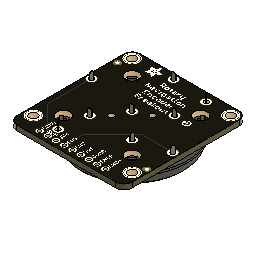
5221 ANO Rotary Encoder (Autodesk Fusion 360 design; units mm, degrees)
part number: MOUNTINGHOLE2.5
part number: FIDUCIAL_1MM
part number: ENCODER_ANO
Autodesk Fusion 360 part; units mm, degrees
sketch "sketch 280" plane through (0, 0, 0) normal (0, 0, 1) x (1, 0, 0)
  line L0 (17.78, -17.78) -> (17.78, 15.24)
  arc A0 (17.78, 15.24) -> (15.24, 17.78) centre (15.24, 15.24) ccw
  line L1 (15.24, 17.78) -> (-15.24, 17.78)
  arc A1 (-15.24, 17.78) -> (-17.78, 15.24) centre (-15.24, 15.24) ccw
  line L2 (-17.78, 15.24) -> (-17.78, -17.78)
  arc A2 (-17.78, -17.78) -> (-15.24, -20.32) centre (-15.24, -17.78) ccw
  line L3 (-15.24, -20.32) -> (15.24, -20.32)
  arc A3 (15.24, -20.32) -> (17.78, -17.78) centre (15.24, -17.78) ccw
extrude "Board" add sketch "sketch 280" along normal blind 1.57 makes body 1 in component "Board"
sketch "sketch 711" plane through (0, 0, 0) normal (0, 0, 1) x (1, 0, 0)
  line L0 (-2, -2) -> (2, -2)
  line L1 (2, -2) -> (2, 2)
  line L2 (2, 2) -> (-2, 2)
  line L3 (-2, 2) -> (-2, -2)
extrude "MOUNTINGHOLE_2.5_PLATED" add sketch "sketch 711" along normal blind 0.1 separate body makes body 2 in component "MOUNTINGHOLE_2.5_PLATED"
sketch "sketch 850" plane through (0, 0, 0) normal (0, 0, 1) x (1, 0, 0)
  line L0 (-0.75, -0.75) -> (0.75, -0.75)
  line L1 (0.75, -0.75) -> (0.75, 0.75)
  line L2 (0.75, 0.75) -> (-0.75, 0.75)
  line L3 (-0.75, 0.75) -> (-0.75, -0.75)
extrude "FIDUCIAL_1MM" add sketch "sketch 850" along normal blind 0.1 separate body makes body 3 in component "FIDUCIAL_1MM"
sketch "sketch 981" plane through (0, 0, 0) normal (0, 0, 1) x (1, 0, 0)
  line L0 (0.016, 0.016) -> (3.794, 0.016)
  line L1 (3.794, 0.016) -> (3.794, 3.794)
  line L2 (3.794, 3.794) -> (0.016, 3.794)
  line L3 (0.016, 3.794) -> (0.016, 0.016)
extrude "ADAFRUIT_3.5MM" add sketch "sketch 981" along normal blind 0.1 separate body makes body 4 in component "ADAFRUIT_3.5MM"
sketch "sketch 1112" plane through (0, 0, 0) normal (0, 0, 1) x (1, 0, 0)
  line L0 (-0.898, -0.898) -> (0.898, -0.898)
  line L1 (0.898, -0.898) -> (0.898, 0.898)
  line L2 (0.898, 0.898) -> (-0.898, 0.898)
  line L3 (-0.898, 0.898) -> (-0.898, -0.898)
extrude "PCBFEAT-REV-040" add sketch "sketch 1112" along normal blind 0.1 separate body makes body 5 in component "PCBFEAT-REV-040"
sketch "sketch 1243" plane through (0, 0, 0) normal (0, 0, 1) x (1, 0, 0)
  line L0 (-17.2, -17.2) -> (17.2, -17.2)
  line L1 (17.2, -17.2) -> (17.2, 17.2)
  line L2 (17.2, 17.2) -> (-17.2, 17.2)
  line L3 (-17.2, 17.2) -> (-17.2, -17.2)
extrude "ENCODER_ANO" add sketch "sketch 1243" along normal blind 0.1 separate body makes body 6 in component "ENCODER_ANO"
sketch "sketch 1374" plane through (0, 0, 0) normal (0, 0, 1) x (1, 0, 0)
  line L0 (-11.43, -0.635) -> (10.66, -0.635)
  line L1 (10.66, -0.635) -> (10.66, 0.635)
  line L2 (10.66, 0.635) -> (-11.43, 0.635)
  line L3 (-11.43, 0.635) -> (-11.43, -0.635)
extrude "1X09_ROUND_70" add sketch "sketch 1374" along normal blind 0.1 separate body makes body 7 in component "1X09_ROUND_70"
sketch "sketch 408" plane through (0, 0, 0) normal (0, 0, 1) x (1, 0, 0)
  circle A0 centre (15.24, -15.24) radius 1.25
  circle A1 centre (-15.24, -15.24) radius 1.25
  circle A2 centre (15.24, 15.24) radius 1.25
  circle A3 centre (-15.24, 15.24) radius 1.25
  circle A4 centre (-1.1102, 1.1102) radius 0.7
  circle A5 centre (-3.182, -3.182) radius 0.8
  circle A6 centre (3.182, 3.182) radius 0.8
  circle A7 centre (-6.5478, -6.5478) radius 0.7
  circle A8 centre (6.5478, 6.5478) radius 0.7
  circle A9 centre (-10.6066, -10.6066) radius 2
  circle A10 centre (10.6066, 10.6066) radius 2
  circle A11 centre (-10.6066, 10.6066) radius 2
  circle A12 centre (10.6066, -10.6066) radius 2
  circle A13 centre (6.5478, -6.5478) radius 0.7
  circle A14 centre (16.1503, -3.6062) radius 0.7
  circle A15 centre (-7.7499, -15.1038) radius 0.7
  circle A16 centre (7.7499, 15.1038) radius 0.7
  circle A17 centre (-3.2527, 16.0796) radius 0.7
  circle A18 centre (-16.1503, 3.6062) radius 0.7
  circle A19 centre (10.16, -18.415) radius 0.5
  circle A20 centre (7.62, -18.415) radius 0.5
  circle A21 centre (5.08, -18.415) radius 0.5
  circle A22 centre (2.54, -18.415) radius 0.5
  circle A23 centre (0, -18.415) radius 0.5
  circle A24 centre (-2.54, -18.415) radius 0.5
  circle A25 centre (-5.08, -18.415) radius 0.5
  circle A26 centre (-7.62, -18.415) radius 0.5
  circle A27 centre (-10.16, -18.415) radius 0.5
extrude "Extrude2" cut sketch "sketch 408" along normal blind 1.57 bodies 1 in component "Board"
sketch "pins" plane through (0, 0, 0) normal (0, 0, 1) x (1, 0, 0) in component "Encoder"
  circle A0 centre (7.7499, 15.1038) radius 0.7
  circle A1 centre (-3.2527, 16.0796) radius 0.7
  circle A2 centre (6.5478, 6.5478) radius 0.7
  circle A3 centre (-1.1102, 1.1102) radius 0.7
  circle A4 centre (-16.1503, 3.6062) radius 0.7
  circle A5 centre (-6.5478, -6.5478) radius 0.7
  circle A6 centre (-7.7499, -15.1038) radius 0.7
  circle A7 centre (16.1503, -3.6062) radius 0.7
  circle A8 centre (6.5478, -6.5478) radius 0.7
  line L0 (-3.9455, 16.1796) -> (-2.5599, 16.1796)
  line L1 (-3.9455, 15.9796) -> (-2.5599, 15.9796)
  line L2 (7.3113, 15.6494) -> (8.3248, 14.7045)
  line L3 (7.1749, 15.5031) -> (8.1885, 14.5582)
  line L4 (-16.2503, 4.2991) -> (-16.2503, 2.9134)
  line L5 (-16.0503, 4.2991) -> (-16.0503, 2.9134)
  line L6 (-1.803, 1.2102) -> (-0.4173, 1.2102)
  line L7 (-0.4173, 1.0102) -> (-1.803, 1.0102)
  line L8 (-7.2406, -6.4478) -> (-5.855, -6.4478)
  line L9 (-5.855, -6.6478) -> (-7.2406, -6.6478)
  line L10 (6.6478, -5.855) -> (6.6478, -7.2406)
  line L11 (6.4478, -5.855) -> (6.4478, -7.2406)
  line L12 (5.855, 6.6478) -> (7.2406, 6.6478)
  line L13 (5.855, 6.4478) -> (7.2406, 6.4478)
  line L14 (16.2503, -2.9134) -> (16.2503, -4.2991)
  line L15 (16.0503, -2.9134) -> (16.0503, -4.2991)
  line L16 (-8.1388, -14.5217) -> (-7.2123, -15.5521)
  line L17 (-8.2875, -14.6555) -> (-7.361, -15.6859)
  line L18 (16.2503, -4.2562) -> (16.0503, -4.2562)
  line L19 (16.2503, -2.9562) -> (16.0503, -2.9562)
  line L20 (6.6478, -7.1978) -> (6.4478, -7.1978)
  line L21 (6.6478, -5.8978) -> (6.4478, -5.8978)
  line L22 (-7.3897, -15.654) -> (-7.2409, -15.5203)
  line L23 (-8.2588, -14.6873) -> (-8.1101, -14.5536)
  line L24 (-7.1978, -6.6478) -> (-7.1978, -6.4478)
  line L25 (-5.8978, -6.6478) -> (-5.8978, -6.4478)
  line L26 (-0.4602, 1.0102) -> (-0.4602, 1.2102)
  line L27 (-1.7602, 1.0102) -> (-1.7602, 1.2102)
  line L28 (-16.0503, 2.9562) -> (-16.2503, 2.9562)
  line L29 (-16.2503, 4.2562) -> (-16.0503, 4.2562)
  line L30 (7.1978, 6.4478) -> (7.1978, 6.6478)
  line L31 (5.8978, 6.4478) -> (5.8978, 6.6478)
  line L32 (8.1571, 14.5874) -> (8.2935, 14.7337)
  line L33 (7.2063, 15.4739) -> (7.3426, 15.6202)
  line L34 (-3.9027, 15.9796) -> (-3.9027, 16.1796)
  line L35 (-2.6027, 15.9796) -> (-2.6027, 16.1796)
  dimension "d70" = 0.1
  dimension "d71" = 0.2
  dimension "d72" = 0.1
  dimension "d73" = 0.2
  dimension "d74" = 0.1
  dimension "d75" = 0.2
  dimension "d76" = 0.1
  dimension "d77" = 0.2
  dimension "d79" = 0.1
  dimension "d80" = 0.2
  dimension "d81" = 0.1
  dimension "d82" = 0.2
  dimension "d83" = 0.1
  dimension "d84" = 0.2
  dimension "d85" = 0.1
  dimension "d86" = 0.2
  dimension "d87" = 0.1
  dimension "d88" = 0.2
  dimension "d91" = 0.65
  dimension "d92" = 0.65
  dimension "d93" = 0.65
  dimension "d94" = 0.65
  dimension "d95" = 0.65
  dimension "d96" = 0.65
  dimension "d97" = 0.65
  dimension "d98" = 0.65
  dimension "d99" = 0.65
  dimension "d100" = 0.65
  dimension "d101" = 0.65
  dimension "d102" = 0.65
  dimension "d103" = 0.65
  dimension "d104" = 0.65
  dimension "d105" = 0.65
  dimension "d106" = 0.65
  dimension "d107" = 0.65
  dimension "d108" = 0.65
  constraint coincident A1 L0.start
  constraint coincident A1 L0.end
  constraint horizontal L0
  constraint coincident A1 L1.start
  constraint coincident A1 L1.end
  constraint horizontal L1
  constraint coincident A0 L2.start
  constraint coincident A0 L2.end
  constraint coincident A0 L3.start
  constraint coincident A0 L3.end
  constraint parallel L2 L3
  constraint coincident A4 L4.start
  constraint coincident A4 L4.end
  constraint vertical L4
  constraint coincident A4 L5.start
  constraint coincident A4 L5.end
  constraint vertical L5
  constraint coincident A3 L6.start
  constraint coincident A3 L6.end
  constraint horizontal L6
  constraint coincident A3 L7.start
  constraint coincident A3 L7.end
  constraint horizontal L7
  constraint coincident A5 L8.start
  constraint coincident A5 L8.end
  constraint horizontal L8
  constraint coincident A5 L9.start
  constraint coincident A5 L9.end
  constraint parallel L8 L9
  constraint coincident A8 L10.start
  constraint coincident A8 L10.end
  constraint vertical L10
  constraint coincident A8 L11.start
  constraint coincident A8 L11.end
  constraint parallel L10 L11
  constraint coincident A2 L12.start
  constraint coincident A2 L12.end
  constraint horizontal L12
  constraint coincident A2 L13.start
  constraint coincident A2 L13.end
  constraint horizontal L13
  constraint coincident A7 L14.start
  constraint coincident A7 L14.end
  constraint vertical L14
  constraint coincident A7 L15.start
  constraint coincident A7 L15.end
  constraint parallel L14 L15
  constraint coincident A6 L16.start
  constraint coincident A6 L16.end
  constraint coincident A6 L17.start
  constraint coincident A6 L17.end
  constraint parallel L16 L17
  constraint coincident L14 L18.start
  constraint coincident L15 L18.end
  constraint perpendicular L15 L18
  constraint coincident L14 L19.start
  constraint coincident L15 L19.end
  constraint perpendicular L15 L19
  constraint coincident L10 L20.start
  constraint coincident L11 L20.end
  constraint perpendicular L11 L20
  constraint coincident L10 L21.start
  constraint coincident L11 L21.end
  constraint perpendicular L11 L21
  constraint coincident L17 L22.start
  constraint coincident L16 L22.end
  constraint perpendicular L16 L22
  constraint coincident L17 L23.start
  constraint coincident L16 L23.end
  constraint perpendicular L16 L23
  constraint coincident L9 L24.start
  constraint coincident L8 L24.end
  constraint perpendicular L8 L24
  constraint coincident L9 L25.start
  constraint perpendicular L9 L25
  constraint coincident L8 L25.end
  constraint coincident L7 L26.start
  constraint coincident L6 L26.end
  constraint perpendicular L6 L26
  constraint coincident L7 L27.start
  constraint coincident L6 L27.end
  constraint perpendicular L6 L27
  constraint coincident L5 L28.start
  constraint coincident L4 L28.end
  constraint perpendicular L4 L28
  constraint coincident L4 L29.start
  constraint coincident L5 L29.end
  constraint perpendicular L5 L29
  constraint coincident L13 L30.start
  constraint coincident L12 L30.end
  constraint perpendicular L12 L30
  constraint coincident L13 L31.start
  constraint coincident L12 L31.end
  constraint perpendicular L12 L31
  constraint coincident L3 L32.start
  constraint coincident L2 L32.end
  constraint perpendicular L2 L32
  constraint coincident L3 L33.start
  constraint coincident L2 L33.end
  constraint perpendicular L2 L33
  constraint coincident L1 L34.start
  constraint coincident L0 L34.end
  constraint perpendicular L0 L34
  constraint coincident L1 L35.start
  constraint coincident L0 L35.end
  constraint perpendicular L0 L35
  measures "d70" distance of A1.centre L0
  measures "d71" distance of L0 L1
  measures "d72" distance of A0.centre L2
  measures "d73" distance of L2 L3
  measures "d74" distance of A4.centre L4
  measures "d75" distance of L4 L5
  measures "d76" distance of A3.centre L6
  measures "d77" distance of L6 L7
  measures "d79" distance of A5.centre L8
  measures "d80" distance of L8 L9
  measures "d81" distance of A8.centre L10
  measures "d82" distance of L10 L11
  measures "d83" distance of A2.centre L12
  measures "d84" distance of L12 L13
  measures "d85" distance of A7.centre L14
  measures "d86" distance of L14 L15
  measures "d87" distance of A6.centre L16
  measures "d88" distance of L16 L17
  measures "d91" distance of A7.centre L18
  measures "d92" distance of A7.centre L19
  measures "d93" distance of A8.centre L20
  measures "d94" distance of A8.centre L21
  measures "d95" distance of A6.centre L22
  measures "d96" distance of A6.centre L23
  measures "d97" distance of A5.centre L24
  measures "d98" distance of A5.centre L25
  measures "d99" distance of A3.centre L27
  measures "d100" distance of A3.centre L26
  measures "d101" distance of A4.centre L29
  measures "d102" distance of A4.centre L28
  measures "d103" distance of A2.centre L31
  measures "d104" distance of A2.centre L30
  measures "d105" distance of A0.centre L32
  measures "d106" distance of A0.centre L33
  measures "d107" distance of A1.centre L34
  measures "d108" distance of A1.centre L35
sketch "circles" plane through (0, 0, 0) normal (0, 0, -1) x (1, 0, 0) in component "Encoder"
  circle A0 centre (0, 0) radius 15.85
  circle A1 centre (0, 0) radius 4
  circle A2 centre (0, 0) radius 11.5
  circle A3 centre (0, 0) radius 17
  dimension "d18" = 31.7
  dimension "d19" = 8
  dimension "d20" = 23
  dimension "d21" = 34
  constraint coincident A0.centre A1.centre
  constraint concentric A0 A2
  constraint concentric A0 A3
  measures "d18" diameter of A0
  measures "d19" diameter of A1
  measures "d20" diameter of A2
  measures "d21" diameter of A3
extrude "Extrude1" add sketch "circles" along normal blind 0.6 from surface at 2 separate body contours A0 | A1 | A2 | A3 makes body 8 in component "Encoder"
extrude "Extrude2'" add sketch "circles" along normal blind 3 from surface at 2.6 separate body contours A0 makes body 9 in component "Encoder"
extrude "Extrude5" add sketch "circles" along normal blind 3 from surface at 2.6 separate body contours A2 makes body 10 in component "Encoder"
extrude "Extrude6" add sketch "circles" along normal blind 3 from surface at 2.6 separate body contours A1 makes body 11 in component "Encoder"
sketch "revolve cut" plane through (0, 0, 0) normal (1, 0, 0) x (0, 1, 0) in component "Encoder"
  line L0 (-15.85, -5.6) -> (15.85, -5.6)
  line L1 (0, 0) -> (0, -5.6)
  line L2 (-11.5, -5.6) -> (-11.5, -5.2)
  line L3 (-11.5, -5.2) -> (-15.45, -5.6)
  dimension "d39" = 0.4
  dimension "d40" = 4.35
  dimension "d41" = 0.4
  constraint coincident L1.start origin
  constraint midpoint L0 L1.end
  constraint coincident L0 L2.start
  constraint perpendicular L0 L2
  constraint coincident L0 L3.end
  measures "d39" distance of L0.start L3.end
  measures "d40" distance of L0.start L2.start
  measures "d41" distance of L2.start L2.end
revolve "Revolve1" cut sketch "revolve cut" angle 360 about axis through (0, 0, 0) along (0, 0, -1) bodies 9 in component "Encoder"
fillet "Fillet1" radius 0.4 2 edges at (-10.7218, 4.1586, -5.6) (-3.7293, -1.4465, -5.6) on bodies 10 in component "Encoder"
fillet "Fillet2" radius 0.4 1 edges at (-3.7293, 1.4465, -5.6) on bodies 11 in component "Encoder"
fillet "Fillet3" radius 0.4 1 edges at (-14.7774, 5.7316, -5.6) on bodies 9 in component "Encoder"
sketch "arrows" plane through (0, 0, -5.6) normal (0, 0, -1) x (1, 0, 0) in component "Encoder"
  line L0 (0, -14.5606) -> (0.75, -12.5)
  line L1 (0.75, -12.5) -> (-0.75, -12.5)
  line L2 (-0.75, -12.5) -> (0, -14.5606)
  line L3 (0, -14.5606) -> (0, -12.5) construction
  dimension "d49" = 1.5
  dimension "d50" = 70
  dimension "d51" = 70
  dimension "d52" = 12.5
  constraint horizontal L1
  constraint midpoint L1 L3.end
  constraint coincident origin L3
  measures "d49" distance of L0.end L1.end
  measures "d50" angle of L0 L1
  measures "d51" angle of L1 L2
  measures "d52" distance of origin L1
extrude "Extrude7" cut sketch "arrows" against normal blind 0.25 from the near side of the face at (14.1333, 0, -5.4667) on bodies 9 bodies 9 in component "Encoder"
pattern_circular "C-Pattern1" count 4 over 360 about axis through (0, 0, 1.75) along (0, 0, 1) of "Extrude7" in component "Encoder"
sketch "dots" plane through (0, 0, -5.6) normal (0, 0, -1) x (1, 0, 0) in component "Encoder"
  circle A0 centre (0, -9) radius 0.5
  line L0 (0, -9) -> (0, 0) construction
  dimension "d57" = 1
  dimension "d58" = 9
  constraint coincident A0.centre L0.start
  constraint coincident L0.end origin
  constraint vertical L0
  measures "d57" diameter of A0
  measures "d58" distance of A0.centre L0.end
extrude "Extrude8" add sketch "dots" along normal blind 0.2 bodies 10 in component "Encoder"
fillet "Fillet4" radius 0.2 1 edges at (-0.4662, 9.1808, -5.8) on bodies 10 in component "Encoder"
pattern_circular "C-Pattern2" count 16 over 360 about axis through (0, 0, 1.75) along (0, 0, 1) of "Extrude8", "Fillet4" in component "Encoder"
extrude "Extrude10" add sketch "pins" along normal blind 3.57 and the other way blind 1 separate body contours L2 L3 L32 L33 | L0 L1 L34 L35 | L12 L13 L30 L31 | L6 L7 L26 L27 | L4 L5 L28 L29 | L8 L9 L24 L25 | L16 L17 L22 L23 | L14 L15 L18 L19 | L10 L11 L20 L21 makes body 12 at (6.6478, -6.7645, 2.0467) makes body 13 at (-16.0503, 3.3896, 2.0467) makes body 14 at (-3.4694, 15.9796, 0.5233) makes body 15 at (16.2503, -3.8229, 2.0467) makes body 16 at (-6.3311, -6.6478, 0.5233) makes body 17 at (6.3311, 6.4478, 0.5233) makes body 18 at (7.9766, 15.0292, 2.0467) makes body 19 at (-0.8935, 1.0102, 0.5233) makes body 20 at (-7.6794, -15.3318, 2.0467) in component "Encoder"
fillet "Fillet5" radius 0.65 18 edges at (6.5478, -5.8978, 3.57) (6.5478, -7.1978, 3.57) (-16.1503, 2.9562, 3.57) (-16.1503, 4.2562, 3.57) (-3.9027, 16.0796, 3.57) (-2.6027, 16.0796, 3.57) (16.1503, -4.2562, 3.57) (16.1503, -2.9562, 3.57) (-5.8978, -6.5478, 3.57) (-7.1978, -6.5478, 3.57) (7.1978, 6.5478, 3.57) (5.8978, 6.5478, 3.57) (7.2744, 15.547, 3.57) (8.2253, 14.6606, 3.57) (-1.7602, 1.1102, 3.57) (-0.4602, 1.1102, 3.57) (-7.3153, -15.5872, 3.57) (-8.1845, -14.6204, 3.57) on bodies 12 13 14 15 16 17 18 19 20 in component "Encoder"
sketch "Sketch6" plane through (0, 0, 0) normal (0, 0, -1) x (1, 0, 0) in component "Encoder"
  line L0 (-16, -6.6274) -> (-6.6274, -16)
  line L1 (-6.6274, -16) -> (6.6274, -16)
  line L2 (6.6274, -16) -> (16, -6.6274)
  line L3 (16, -6.6274) -> (16, 6.6274)
  line L4 (16, 6.6274) -> (6.6274, 16)
  line L5 (6.6274, 16) -> (-6.6274, 16)
  line L6 (-6.6274, 16) -> (-16, 6.6274)
  line L7 (-16, 6.6274) -> (-16, -6.6274)
  dimension "d113" = 32
  constraint horizontal L1
  measures "d113" distance of L3 L7
extrude "Extrude11" add sketch "Sketch6" along normal blind 1.4 separate body makes body 21 in component "Encoder"
extrude "Extrude12" add sketch "circles" along normal blind 0.6 from surface at 1.4 contours A0 | A1 | A2 bodies 21 in component "Encoder"
sketch "Sketch7" plane through (0, 0, 0) normal (0, 0, -1) x (1, 0, 0) in component "Encoder"
  circle A0 centre (-10.6066, -10.6066) radius 2
  circle A1 centre (10.6066, -10.6066) radius 2
  circle A2 centre (10.6066, 10.6066) radius 2
  circle A3 centre (-10.6066, 10.6066) radius 2
  line L0 (-10.7834, 9.3692) -> (-11.844, 10.4298)
  line L1 (-11.844, 10.4298) -> (-10.4298, 11.844)
  line L2 (-10.4298, 11.844) -> (-9.3692, 10.7834)
  line L3 (-9.3692, 10.7834) -> (-10.7834, 9.3692)
  line L4 (-11.3137, 9.8995) -> (-10.6066, 10.6066)
  line L5 (-10.6066, 10.6066) -> (-10.0763, 10.0763) construction
  line L6 (-10.6066, 10.6066) -> (-10.6066, 11.4116) construction
  line L7 (-9.8995, 11.3137) -> (-10.6066, 10.6066)
  dimension "d133" = 1.5
  dimension "d134" = 2
  dimension "d135" = 135
  constraint perpendicular L0 L1
  constraint perpendicular L1 L2
  constraint perpendicular L2 L3
  constraint coincident L0.start L3.end
  constraint midpoint L0 L4.start
  constraint perpendicular L0 L4
  constraint perpendicular L4 L5
  constraint midpoint L3 L5.end
  constraint coincident A3.centre L4.end
  constraint vertical L6
  constraint midpoint L2 L7.start
  measures "d133" distance of L0.start L0.end
  measures "d134" distance of L2.end L0.start
  measures "d135" angle of L4 L6
extrude "Extrude13" cut sketch "Sketch7" along normal blind 0.5 contours L0 L2 L3 L4 L7 bodies 21 in component "Encoder"
extrude "Extrude14" add sketch "Sketch7" against normal blind 1 contours L0 L1 L2 L4 L7 bodies 21 in component "Encoder"
pattern_circular "C-Pattern3" count 4 over 360 about axis through (0, 0, 1.75) along (0, 0, 1) of "Extrude13", "Extrude14" in component "Encoder"
component "Board" placed x (1, 0, 0) y (0, 1, 0) z (0, 0, 1) at (0, 0, 0)
component "MOUNTINGHOLE_2.5_PLATED" placed x (-1, 0, 0) y (0, -1, 0) z (0, 0, 1) at (15.24, -15.24, 1.57)
component "MOUNTINGHOLE_2.5_PLATED" placed x (-1, 0, 0) y (0, -1, 0) z (0, 0, 1) at (-15.24, -15.24, 1.57)
component "MOUNTINGHOLE_2.5_PLATED" placed x (-1, 0, 0) y (0, -1, 0) z (0, 0, 1) at (15.24, 15.24, 1.57)
component "MOUNTINGHOLE_2.5_PLATED" placed x (-1, 0, 0) y (0, -1, 0) z (0, 0, 1) at (-15.24, 15.24, 1.57)
component "FIDUCIAL_1MM" placed x (-1, 0, 0) y (0, -1, 0) z (0, 0, 1) at (-16.383, 11.874, 1.57)
component "FIDUCIAL_1MM" placed x (-1, 0, 0) y (0, -1, 0) z (0, 0, 1) at (16.637, -12.103, 1.57)
component "ADAFRUIT_3.5MM" placed x (1, 0, 0) y (0, 1, 0) z (0, 0, 1) at (-10.16, 13.335, 1.57)
component "PCBFEAT-REV-040" placed x (-1, 0, 0) y (0, -1, 0) z (0, 0, 1) at (10.541, 6.35, 1.57)
component "ENCODER_ANO" placed x (0.707107, -0.707107, 0) y (-0.707107, -0.707107, 0) z (0, 0, -1) at (0, 0, 0)
component "1X09_ROUND_70" placed x (-1, 0, 0) y (0, -1, 0) z (0, 0, 1) at (0, -18.415, 1.57)
component "Encoder" placed x (1, 0, 0) y (0, 1, 0) z (0, 0, 1) at (0, 0, 0)
equation "d112 = ( 1.3 / 2 ) * 1 mm"
named bodies: "Board", "MOUNTINGHOLE_2.5_PLATED", "FIDUCIAL_1MM", "ADAFRUIT_3.5MM", "PCBFEAT-REV-040", "ENCODER_ANO", "1X09_ROUND_70", "base", "directions", "wheel", "center button"
